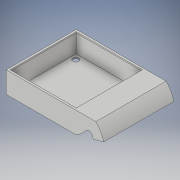
# Autodesk Inventor part: fan_shourd
Saved by Autodesk Inventor 2019 (Build 230136000, 136)
## iProperties
Created: 2020-03-22
Part Number: fan_shourd
Material: Generisch
Document SubType Name: Modeling
Designer: marc
Density: 1 g/cm^3
Appearance: Vorgabe
Author: marc
## iProperties of the stored document fan_shourd_3D-Druck.ipt
Created: 2020-03-22
Part Number: fan_shourd_3D-Druck
Material: Generisch
Document SubType Name: Modeling
Designer: marc
Density: 1 g/cm^3
Appearance: Vorgabe
Author: marc
Autodesk Inventor part; units mm, degrees
ref_plane "YZ Plane" through (0, 0, 0) normal (1, 0, 0) x (0, 1, 0)
ref_plane "XZ Plane" through (0, 0, 0) normal (0, 1, 0) x (-1, 0, 0)
ref_plane "XY Plane" through (0, 0, 0) normal (0, 0, 1) x (1, 0, 0)
sketch "Skizze1" plane through (0, 0, 0) normal (0, 1, 0) x (-1, 0, 0)
  line L0 (0, 0) -> (43, 0)
  line L1 (43, 0) -> (43, 43)
  line L2 (43, 43) -> (0, 43)
  line L3 (0, 43) -> (0, 0)
  line L4 (41.75, 41.75) -> (-1.25, 41.75)
  line L5 (-1.25, 41.75) -> (-1.25, -1.25)
  line L6 (-1.25, -1.25) -> (41.75, -1.25)
  line L7 (41.75, -1.25) -> (41.75, 41.75)
  dimension "d0" = 43
  dimension "d1" = 43
  dimension "d2" = 43
  dimension "d3" = 43
  dimension "d4" = 1.25
  dimension "d5" = 1.25
  constraints: 16 end point, 4 parallel, 2 horizontal, 2 perpendicular
  measures "d0" distance of L2.end L1.end
  measures "d1" distance of L1.end L0.end
  measures "d2" distance of L6.end L5.end
  measures "d3" distance of L5.end L4.end
  measures "d4" distance between parallel lines of L2 L4
  measures "d5" distance between parallel lines of L1 L7
extrude "Extrusion1" add sketch "Skizze1" along normal blind 13 contours L3 L4 L7 L0 | L0 L7 L6 L5 L4 L3
shell "Wandung1" thickness 0.75 removed faces 1 at (1.25, 4.3333, 27.4167)
shell "Wandung2" thickness 1.25 removed faces 2 at (-13.0833, 13, 13.0833) at (-12.8333, 12.25, 13.3333)
sketch "Skizze2" plane through (-40.5, 0.75, 40.5) normal (0, 1, 0) x (1, 0, 0)
  line L0 (0, 40.5) -> (40.5, 40.5) projected
  line L1 (40.5, 0) -> (0, 0) projected
  line L2 (0, 0) -> (0, 40.5) projected
  point P0 (40.5, 40.5)
  point P1 (2.5, 2.75)
  point P2 (2.5, 37.75)
  point P3 (37.5, 2.75)
  point P4 (37.5, 37.75)
  dimension "d10" = 35
  dimension "d11" = 2.75
  dimension "d12" = 2.75
  dimension "d13" = 2.5
  dimension "d14" = 35
  constraints: 2 horizontal alignment, 2 vertical alignment
  measures "d10" distance of point (2.5, 37.75) point (2.5, 2.75)
  measures "d11" distance from line of L0 point (2.5, 37.75)
  measures "d12" distance from line of L1 point (2.5, 2.75)
  measures "d13" distance from line of L2 point (2.5, 2.75)
  measures "d14" distance of point (37.5, 2.75) point (2.5, 2.75)
hole "Bohrung1" at (-38, 0.75, 37.75) at (-38, 0.75, 2.75) at (-3, 0.75, 37.75) at (-3, 0.75, 2.75) direction (0, -1, 0) diameter 3.6 end through all clearance for "Flachkopfsenkschraube DIN EN ISO 2009" size "M3" standard "DIN"
move faces "Verschieben1" translate (14, 0, 0) faces at (1.25, 0.25, 27.1667)
sketch "Skizze3" plane through (-41.75, 0, 41.75) normal (0, 0, 1) x (1, 0, 0)
  line L0 (0, 0) -> (57, 0) projected
  line L1 (57, 0) -> (57, 13) projected
  line L2 (55, 13) -> (42, 0)
  line L3 (0, 13) -> (57, 13) projected
  point P0 (41.75, 0)
  dimension "d47" = 2
  dimension "d48" = 45
  constraints: 2 end point, 2 point on line
  measures "d47" distance from line of L1 L2.start
  measures "d48" angle of L3 L2
extrude "Extrusion2" cut sketch "Skizze3" against normal up to surface (43 mm away)
sketch "Skizze4" plane through (13.25, 13, 41.75) normal (0.7071068, -0.7071068, 0) x (-0.7071068, -0.7071068, 0)
  line L0 (18.3848, 43) -> (18.3848, 0) projected
  line L1 (18.3848, 0) -> (0, 0) projected
  line L2 (18.3848, 43) -> (5.3848, 43)
  line L3 (5.3848, 43) -> (5.3848, 0)
  line L4 (5.3848, 0) -> (18.3848, 0)
  line L5 (18.3848, 0) -> (18.3848, 43)
  point P0 (18.5616, 41.75)
  dimension "d29" = 13
  constraints: 8 end point, 2 parallel, 1 horizontal, 1 perpendicular, 1 point on line
  measures "d29" distance between parallel lines of L0 L3
extrude "Extrusion3" add sketch "Skizze4" along normal blind 1.25
fillet "Rundung1" radius 6.25 2 edges at (1.1339, -0.8839, 20.25) (1, 0.75, 20.25)
sketch "Skizze6" plane through (13.25, 13, 41.75) normal (0.7071068, -0.7071068, 0) x (-0.7071068, -0.7071068, 0)
  line L0 (5.3848, 0) -> (5.3848, 0.75) projected
  line L1 (0, 43) -> (5.3848, 43) projected
  line L2 (0, 0) -> (0, 43) projected
  line L3 (5.3848, 0) -> (0, 0) projected
  line L4 (5.3848, 42.25) -> (5.3848, 43) projected
  line L5 (1.0607, 42.25) -> (1.0607, 0.75) projected
  line L6 (18.5616, 51.6) -> (18.5616, -8.6) projected
  line L7 (1.0607, 0.75) -> (5.3848, 0.75) projected
  line L8 (5.3848, 42.25) -> (1.0607, 42.25) projected
  point P0 (18.5616, 41.75)
revolve "Umdrehung1" add sketch "Skizze6" angle 30 about axis through (0.125, -0.125, -10) along (0, 0, -1)
fillet "Rundung2" radius 1.75 1 edges at (9.4424, 9.1924, 20.25)
sketch "Skizze8" plane through (-41.75, 0, 41.75) normal (0, 0, 1) x (1, 0, 0)
  line L0 (58.7796, 4.4046) -> (54.6028, 3.2854) projected
  line L1 (54.6028, 3.2854) -> (53.3954, 2.9619)
  line L2 (52.0343, 8.2665) -> (52.0763, 8.3085) projected
  line L3 (52.0343, 8.2665) -> (51.1459, 7.3782)
  arc A0 (53.3954, 2.9619) -> (51.1459, 7.3782) centre (41.875, -0.125) ccw
  arc A1 (54.6028, 3.2854) -> (52.0343, 8.2665) centre (41.875, -0.125) ccw projected
  line L4 (52.0343, 8.2665) -> (45.5355, 1.7678) projected
  point P0 (41.75, 0)
  dimension "d42" = 1.25
  constraints: 4 end point, 2 collinear, 2 point on circle, 1 centre point, 1 concentric
  measures "d42" distance of L0.end L1.end
extrude "Extrusion5" add sketch "Skizze8" against normal up to surface (43 mm away)
fillet "Rundung3" radius 2 2 edges at (9.3959, 7.3782, 20.25) (10.2843, 8.2665, 20.25)
equation "\"d5\" = d4"
